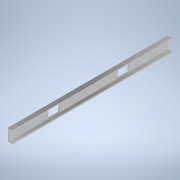
# Autodesk Inventor part: NASA-20-SP-01
Saved by Autodesk Inventor 2020 (Build 240168000, 168)
## iProperties
Created: 2019-09-05
Part Number: NASA-20-SP-01
Material: Aluminum 6061
Description: SIDE PLATE
Document SubType Name: Modeling
Designer: Rick Szalay
Stock Number: 1630T31
Density: 2.7 g/cm^3
Appearance: Aluminum - Flat
Author: Rick Szalay
Autodesk Inventor part; units mm, degrees
ref_plane "YZ Plane" through (0, 0, 0) normal (1, 0, 0) x (0, 1, 0)
ref_plane "XZ Plane" through (0, 0, 0) normal (0, 1, 0) x (-1, 0, 0)
ref_plane "XY Plane" through (0, 0, 0) normal (0, 0, 1) x (1, 0, 0)
sketch "Sketch3" plane through (0, 0, 0) normal (0, 0, 1) x (1, 0, 0)
  line L0 (0, 25.4) -> (0, -25.4)
  line L1 (0, 25.4) -> (19.05, 25.4)
  line L2 (19.05, 25.4) -> (19.05, 22.225)
  line L3 (19.05, 22.225) -> (3.048, 22.225)
  line L4 (3.048, 22.225) -> (3.048, -22.225)
  line L5 (3.048, -22.225) -> (19.05, -22.225)
  line L6 (19.05, -22.225) -> (19.05, -25.4)
  line L7 (19.05, -25.4) -> (0, -25.4)
  line L8 (0, 0) -> (3.048, 0) construction
  dimension "d7" = 50.8
  dimension "d10" = 19.05
  dimension "d33" = 3.175
  dimension "d34" = 16.002
  constraints: 18 end point, 6 perpendicular, 2 horizontal, 2 midpoint, 1 coincident, 1 vertical, 1 other
  measures "d7" distance of L0.start L0.end
  measures "d10" distance of L0.start L1.end
  measures "d33" distance between parallel lines of L3 L1
  measures "d34" distance between parallel lines of L6 L4
extrude "Extrusion3" add sketch "Sketch3" along normal mid plane 660.4
fillet "Fillet1" radius 1.5875 4 edges at (19.05, 22.225, 0) (19.05, -22.225, 0) (3.048, -22.225, 0) (3.048, 22.225, 0)
sketch "Sketch6" plane through (0, -25.4, 330.2) normal (-1, 0, 0) x (0, 0, 1)
  line L0 (-496.189, 3.81) -> (-453.009, 3.81)
  line L1 (-453.009, 3.81) -> (-453.009, 46.99)
  line L2 (-453.009, 46.99) -> (-496.189, 46.99)
  line L3 (-496.189, 46.99) -> (-496.189, 3.81)
  line L4 (-496.189, 3.81) -> (-453.009, 46.99) construction
  line L5 (-453.009, 3.81) -> (-496.189, 46.99) construction
  line L6 (-207.391, 3.81) -> (-164.211, 3.81)
  line L7 (-164.211, 3.81) -> (-164.211, 46.99)
  line L8 (-164.211, 46.99) -> (-207.391, 46.99)
  line L9 (-207.391, 46.99) -> (-207.391, 3.81)
  line L10 (-207.391, 3.81) -> (-164.211, 46.99) construction
  line L11 (-164.211, 3.81) -> (-207.391, 46.99) construction
  point P0 (-330.2, 25.4)
  point P1 (-474.599, 25.4)
  point P2 (-185.801, 25.4)
  point P3 (-474.599, 25.4)
  point P4 (-185.801, 25.4)
  dimension "d35" = 288.798
  dimension "d36" = 144.399
  dimension "d37" = 43.18
  constraints: 24 end point, 6 midpoint, 4 parallel, 4 perpendicular, 2 horizontal, 2 horizontal alignment, 1 point on line
  measures "d35" distance of point (-474.599, 25.4) point (-185.801, 25.4)
  measures "d36" distance of point (-185.801, 25.4) point (-330.2, 25.4)
  measures "d37" distance of L2.end L0.start
extrude "Extrusion4" cut sketch "Sketch6" against normal through all
sketch "Sketch7" plane through (3.048, -20.6375, 330.2) normal (1, 0, 0) x (0, 0, -1)
  circle A0 centre (227.075, 4.7625) radius 2.4194 projected
  circle A1 centre (227.075, 36.5125) radius 2.4194 projected
  circle A2 centre (144.525, 4.7625) radius 2.4194 projected
  circle A3 centre (144.525, 36.5125) radius 2.4194 projected
  circle A4 centre (515.875, 4.7625) radius 2.4194 projected
  circle A5 centre (515.875, 36.5125) radius 2.4194 projected
  circle A6 centre (433.325, 4.7625) radius 2.4194 projected
  circle A7 centre (433.325, 36.5125) radius 2.4194 projected
  point P0 (330.2, 20.6375)
hole "Hole3" at (3.048, -15.875, -185.675) at (3.048, 15.875, -185.675) at (3.048, -15.875, -103.125) at (3.048, 15.875, -103.125) at (3.048, -15.875, 103.125) at (3.048, 15.875, 103.125) at (3.048, -15.875, 185.675) at (3.048, 15.875, 185.675) direction (-1, 0, 0) diameter 6.7564 end through all clearance for "Socket Head Cap Screw" size "1/4" standard "Ansi Unified Screw Threads"
equation "\"d11\" = Length"
equation "\"Length\" = 660.4"
body "Solid2"
